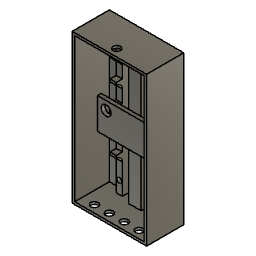
Locker-Button project (Autodesk Fusion 360 design; units mm, degrees)
Autodesk Fusion 360 part; units mm, degrees
note: some values were not read from the file. Chosen so that the rebuilt part matches the saved one: which face or edge a step refers to; where a step ends.
sketch "Schizzo1" plane through (0, 0, 0) normal (0, 1, 0) x (1, 0, 0) in component "Scatola di fissaggio"
  line L0 (-30, -60) -> (30, -60)
  line L1 (30, -60) -> (30, 60)
  line L2 (30, 60) -> (-30, 60)
  line L3 (-30, 60) -> (-30, -60)
  point P0 (0, -60)
  point P1 (-30, 0)
  dimension "d1" = 60
  dimension "d2" = 120
  constraint horizontal L0
  constraint vertical L1
  constraint horizontal L2
  constraint vertical L3
  constraint midpoint L0 P0
  constraint midpoint L3 P1
  constraint vertical origin P0
  constraint horizontal origin P1
  measures "d1" distance of L0.start L0.end
  measures "d2" distance of L0.start L2.end
extrude "Estrusione1" add sketch "Schizzo1" along normal blind 30 makes body 1 in component "Scatola di fissaggio"
shell "Svuotamento1" thickness 2 removed faces 1 at (-10, 0, 20) on bodies 1 in component "Scatola di fissaggio"
ref_plane "Piano di lavoro1" through (0, 14, -58) normal (0, 0, 1) x (1, 0, 0) in component "Guida lineare"
sketch "Schizzo1 (2)" plane through (0, 12.5, -58) normal (0, 0, 1) x (1, 0, 0) in component "Guida lineare"
  line L0 (0, -18.6959) -> (0, 30.9147) construction
  line L1 (0, 8) -> (-5, 8)
  line L2 (-5, 8) -> (-5, 11.5)
  line L3 (-3.5, 13) -> (-2.5, 13)
  line L4 (-2.5, 13) -> (-2.5, 15.5)
  line L5 (28, 15.5) -> (-28, 15.5)
  line L6 (-5, 11.5) -> (-3.5, 13)
  line L7 (0, 8) -> (5, 8)
  line L8 (5, 8) -> (5, 11.5)
  line L9 (5, 11.5) -> (3.5, 13)
  line L10 (3.5, 13) -> (2.5, 13)
  line L11 (2.5, 13) -> (2.5, 15.5)
  point P0 (-5, 13)
  dimension "d7" = 2.5
  dimension "d8" = 5
  dimension "d9" = 5
  dimension "d10" = 2.5
  dimension "d11" = 1.5
  dimension "d12" = 1.5
  constraint vertical L0
  constraint coincident origin L0
  constraint coincident L0 L1.start
  constraint perpendicular L0 L1
  constraint perpendicular L1 L2
  constraint perpendicular L2 L3
  constraint perpendicular L3 L4
  constraint coincident L4.end L5
  constraint coincident P0 L2
  constraint coincident P0 L3
  constraint symmetric L0 L1.start L7.start
  constraint symmetric L0 L1.end L7.end
  constraint symmetric L0 L3.end L10.end
  constraint symmetric L0 L4.end L11.end
  constraint symmetric L0 L2.end L8.end
  constraint symmetric L0 L3.start L9.end
  measures "d7" distance of L3.end L4.end
  measures "d8" distance of L1.end P0
  measures "d9" distance of L1.start L1.end
  measures "d10" distance of L0 L4
  measures "d11" distance of P0 L2.end
  measures "d12" distance of P0 L3.start
extrude "Estrusione1'" add sketch "Schizzo1 (2)" along normal up to near side of body 1 separate body makes body 2 in component "Guida lineare"
sketch "Schizzo5" plane through (0, 0, 0) normal (0, 0, 1) x (1, 0, 0) in component "Base mobile"
  line L0 (5, 24) -> (3.5, 25.5)
  line L1 (5, 20.5) -> (5, 24)
  line L2 (0, 20.5) -> (5, 20.5)
  line L3 (0, 20) -> (5.5, 20)
  line L4 (5.5, 20) -> (5.5, 24.2071)
  line L5 (5.5, 24.2071) -> (3.8536, 25.8536)
  line L6 (3.8536, 25.8536) -> (8.8536, 25.8536)
  line L7 (8.8536, 25.8536) -> (8.8536, 15.8536)
  line L8 (8.8536, 15.8536) -> (0, 15.8536)
  line L9 (0, -6.1959) -> (0, 43.4147)
  line L10 (-8.8536, 15.8536) -> (0, 15.8536)
  line L11 (-8.8536, 25.8536) -> (-8.8536, 15.8536)
  line L12 (0, 20) -> (-5.5, 20)
  line L13 (-5.5, 20) -> (-5.5, 24.2071)
  line L14 (-3.8536, 25.8536) -> (-8.8536, 25.8536)
  line L15 (-5.5, 24.2071) -> (-3.8536, 25.8536)
  dimension "d24" = 0.5
  dimension "d25" = 10
  dimension "d26" = 5
  constraint perpendicular L1 L6
  constraint perpendicular L6 L7
  constraint perpendicular L7 L8
  constraint coincident L8.end L9
  constraint symmetric L3.start L9 L12.start
  constraint symmetric L3.end L9 L12.end
  constraint symmetric L4.end L9 L13.end
  constraint symmetric L5.end L9 L14.start
  constraint symmetric L6.end L9 L11.start
  constraint symmetric L7.end L9 L10.start
  constraint symmetric L8.end L9 L10.end
  measures "d25" distance of L6.end L7.end
  measures "d26" distance of L5.end L6.end
extrude "Estrusione2" add sketch "Schizzo5" along normal blind 5 and the other way blind 5 separate body makes body 3 in component "Base mobile"
sketch "Schizzo6" plane through (0, 15.8536, 0) normal (0, -1, 0) x (1, 0, 0) in component "Base mobile"
  line L0 (8.8536, -5) -> (8.8536, 5)
  line L1 (8.8536, 5) -> (-8.8536, 5)
  line L2 (-8.8536, 5) -> (-8.8536, -5)
  line L3 (-8.8536, -5) -> (8.8536, -5)
  line L4 (22.5, -12.5) -> (-22.5, -12.5)
  line L5 (-22.5, -12.5) -> (-22.5, 12.5)
  line L6 (-22.5, 12.5) -> (22.5, 12.5)
  line L7 (22.5, 12.5) -> (22.5, -12.5)
  point P0 (0, -12.5)
  point P1 (22.5, 0)
  dimension "d31" = 45
  dimension "d32" = 25
  constraint horizontal L4
  constraint vertical L5
  constraint horizontal L6
  constraint vertical L7
  constraint midpoint L4 P0
  constraint midpoint L7 P1
  constraint horizontal origin P1
  constraint vertical origin P0
  measures "d31" distance of L4.start L4.end
  measures "d32" distance of L4.start L6.end
extrude "Estrusione3" add sketch "Schizzo6" along normal blind 3 separate body contours L0 L1 L2 L3 | L4 L5 L6 L7 makes body 4 in component "Base mobile"
sketch "Schizzo1 (3)" plane through (0, 28, 0) normal (0, -1, 0) x (1, 0, 0) in component "cremagliera"
  line L0 (-28, 58) -> (-28, -58)
  line L1 (-28, -58) -> (28, -58)
  line L2 (28, -58) -> (28, 58)
  line L3 (28, 58) -> (-28, 58)
  line L4 (-12.5, -58) -> (-17.5, -58)
  line L5 (-17.5, -58) -> (-17.5, 58)
  line L6 (-17.5, 58) -> (-12.5, 58)
  line L7 (-12.5, 58) -> (-12.5, -58)
  dimension "d35" = 5
  dimension "d36" = 12.5
  constraint horizontal L4
  constraint vertical L5
  constraint horizontal L6
  constraint vertical L7
  constraint collinear L1 L4
  constraint collinear L3 L6
  measures "d35" distance of L4.start L4.end
  measures "d36" distance of origin L7
extrude "Estrusione1''" add sketch "Schizzo1 (3)" along normal blind 10 separate body contours L1 L3 L4 L5 L6 L7 makes body 5 in component "cremagliera"
sketch "Schizzo7" plane through (0, 12.8536, 0) normal (0, -1, 0) x (1, 0, 0) in component "Base mobile"
  line L0 (22.5, 12.5) -> (-22.5, 12.5)
  line L1 (-22.5, 12.5) -> (-22.5, -12.5)
  line L2 (-22.5, -12.5) -> (22.5, -12.5)
  line L3 (22.5, -12.5) -> (22.5, 12.5)
  circle A0 centre (-15.5, 5.5) radius 4
  dimension "d51" = 8
  dimension "d53" = 7
  dimension "d54" = 7
  measures "d51" diameter of A0
  measures "d53" distance of L0 A0.centre
  measures "d54" distance of L1 A0.centre
extrude "Estrusione4" cut sketch "Schizzo7" along normal up to far side of body 4 contours A0 bodies 4 in component "Base mobile"
sketch "Schizzo3" plane through (-17.5, 0, 0) normal (-1, 0, 0) x (0, -1, 0) in component "cremagliera"
  line L0 (-28, 58) -> (-28, -58)
  line L1 (-28, -58) -> (-18, -58)
  line L2 (-18, -58) -> (-18, 58)
  line L3 (-18, 58) -> (-28, 58)
  arc A0 (-18, -29) -> (-23, -34) centre (-18, -34) ccw
  line L4 (-23, -77.8463) -> (-23, -58) construction
  line L5 (-23, -34) -> (-23, 61.2431) construction
  line L6 (-18, -29) -> (-18, -27)
  line L7 (-23, -27) -> (-23, -17)
  line L8 (-18, -27) -> (-23, -27)
  arc A1 (-18, -12) -> (-23, -17) centre (-18, -17) ccw
  line L9 (-18, -12) -> (-18, -10)
  line L10 (-18, -10) -> (-23, -10)
  line L11 (-23, -10) -> (-23, 0)
  arc A2 (-18, 5) -> (-23, 0) centre (-18, 0) ccw
  line L12 (-18, 5) -> (-18, 7)
  line L13 (-23, 7) -> (-18, 7)
  line L14 (-23, 7) -> (-23, 17)
  arc A3 (-18, 22) -> (-23, 17) centre (-18, 17) ccw
  line L15 (-18, 22) -> (-18, 24)
  line L16 (-23, 24) -> (-18, 24)
  line L17 (-23, 24) -> (-23, 34)
  arc A4 (-18, 39) -> (-23, 34) centre (-18, 34) ccw
  line L18 (-18, 39) -> (-18, 41)
  line L19 (-23, 41) -> (-23, 58)
  line L20 (-18, 41) -> (-23, 41)
  line L21 (-23, -34) -> (-23, -58)
  dimension "d57" = 5
  dimension "d58" = 24
  dimension "d59" = 2
  dimension "d60" = 10
  dimension "d61" = 2
  dimension "d62" = 10
  dimension "d63" = 2
  dimension "d64" = 10
  dimension "d65" = 2
  dimension "d66" = 10
  dimension "d67" = 2
  constraint parallel L0 L4
  constraint coincident L2 A0.centre
  constraint tangent A0 L4
  constraint midpoint L1 L4.end
  constraint coincident L2 A0.start
  constraint collinear L4 L5
  constraint coincident L2 L6.end
  constraint parallel L2 L6
  constraint coincident L5 L7.start
  constraint coincident L5 L7.end
  constraint perpendicular L7 L8
  constraint coincident L2 A1.centre
  constraint horizontal L7.end A1.centre
  constraint coincident L2 A1.start
  constraint coincident L2 L9.end
  constraint coincident L5 L10.end
  constraint perpendicular L5 L10
  constraint coincident L5 L11.end
  constraint coincident L2 A2.centre
  constraint horizontal L11.end A2.centre
  constraint coincident L2 A2.start
  constraint coincident L2 L12.end
  constraint parallel L2 L12
  constraint coincident L5 L13.start
  constraint perpendicular L2 L13
  constraint coincident L5 L14.end
  constraint coincident L2 A3.centre
  constraint coincident L14.end A3
  constraint horizontal L14.end A3.centre
  constraint coincident L2 A3.start
  constraint coincident L2 L15.end
  constraint coincident L5 L16.start
  constraint coincident L5 L17.end
  constraint horizontal L16
  constraint coincident L2 A4.centre
  constraint tangent L17 A4
  constraint coincident L2 A4.start
  constraint coincident L2 L18.end
  constraint parallel L2 L18
  constraint coincident L5 L19.start
  constraint midpoint L3 L19.end
  constraint perpendicular L3 L19
  constraint perpendicular L19 L20
  measures "d57" distance of L0 L4
  measures "d58" distance of L1.end A0.centre
  measures "d59" distance of A0.start L6.end
  measures "d60" distance of L7.start L7.end
  measures "d61" distance of A1.start L9.end
  measures "d62" distance of L10.end L11.end
  measures "d63" distance of A2.start L12.end
  measures "d64" distance of L13.start L14.end
  measures "d65" distance of A3.start L15.end
  measures "d66" distance of L16.start L17.end
  measures "d67" distance of A4.start L18.end
extrude "Estrusione3'" cut sketch "Schizzo3" against normal up to surface (5 mm away) contours L2 L3 L19 L20 | L1 L2 A0 L21 | L2 L16 L17 A4 | L2 L7 L8 A1 | L2 L13 L14 A3 | L2 L10 L11 A2 bodies 5 in component "cremagliera"
sketch "Schizzo4" plane through (0, 23, 0) normal (0, -1, 0) x (1, 0, 0) in component "cremagliera"
  line L0 (-12.5, -58) -> (-12.5, -34)
  line L1 (-12.5, -34) -> (-17.5, -34)
  line L2 (-17.5, -34) -> (-17.5, -58)
  line L3 (-17.5, -58) -> (-12.5, -58)
  circle A0 centre (-15, -48) radius 2
  circle A1 centre (-15, 53) radius 2
  line L4 (-17.5, 41) -> (-17.5, 58)
  line L5 (-28, 58) -> (28, 58)
  dimension "d70" = 4
  dimension "d71" = 2.5
  dimension "d72" = 10
  dimension "d73" = 4
  dimension "d74" = 2.5
  dimension "d75" = 5
  measures "d70" diameter of A0
  measures "d71" distance of L2 A0.centre
  measures "d72" distance of L3 A0.centre
  measures "d73" diameter of A1
  measures "d74" distance of A1.centre L4
  measures "d75" distance of A1.centre L5
extrude "Estrusione4'" cut sketch "Schizzo4" against normal up to surface (5 mm away) contours A0 | A1 bodies 5 in component "cremagliera"
sketch "Schizzo2" plane through (0, 0, 0) normal (0, 1, 0) x (1, 0, 0) in component "Scatola di fissaggio"
  circle A0 centre (-15, 48) radius 2
  circle A1 centre (-15, -53) radius 2
extrude "Estrusione2'" cut sketch "Schizzo2" along normal up to surface (30 mm away) bodies 1 in component "Scatola di fissaggio"
sketch "Schizzo3 (2)" plane through (0, 0, 60) normal (0, 0, 1) x (-1, 0, 0) in component "Scatola di fissaggio"
  line L0 (30, 0) -> (-30, 0)
  line L1 (-30, 0) -> (-30, -30)
  line L2 (-30, -30) -> (30, -30)
  line L3 (30, -30) -> (30, 0)
  circle A0 centre (0, -6) radius 3
  dimension "d82" = 6
  dimension "d83" = 6
  constraint vertical origin A0.centre
  measures "d82" diameter of A0
  measures "d83" distance of L0 A0.centre
extrude "Estrusione3''" cut sketch "Schizzo3 (2)" against normal up to surface (2 mm away) contours A0 bodies 1 in component "Scatola di fissaggio"
sketch "Schizzo4 (2)" plane through (0, 0, -60) normal (0, 0, -1) x (1, 0, 0) in component "Scatola di fissaggio"
  line L0 (30, 0) -> (-30, 0)
  line L1 (-30, 0) -> (-30, -30)
  line L2 (-30, -30) -> (30, -30)
  line L3 (30, -30) -> (30, 0)
  circle A0 centre (-18, -6) radius 3
  line L4 (-68.094, -6) -> (66.0156, -6) construction
  line L5 (0, 54.335) -> (0, -66.5386) construction
  circle A1 centre (-6, -6) radius 3
  circle A2 centre (18, -6) radius 3
  circle A3 centre (6, -6) radius 3
  dimension "d86" = 6
  dimension "d91" = 12
  dimension "d92" = 6
  dimension "d93" = 6
  dimension "d94" = 12
  dimension "d97" = 12
  constraint perpendicular L3 L4
  constraint perpendicular L0 L5
  constraint coincident A0.centre L4
  constraint coincident L4 A1.centre
  constraint symmetric A0 L5 A2
  constraint symmetric L5 A1 A3
  measures "d86" diameter of A0
  measures "d91" distance of L1 A0.centre
  measures "d92" distance of L0 L4
  measures "d93" diameter of A1
  measures "d94" distance of A0.centre A1.centre
  measures "d97" distance of L3 A2.centre
extrude "Estrusione4''" cut sketch "Schizzo4 (2)" against normal up to surface (2 mm away) contours A0 | A1 | A2 | A3 bodies 1 in component "Scatola di fissaggio"
component "Scatola di fissaggio" placed x (1, 0, 0) y (0, 1, 0) z (0, 0, 1) at (0, 0, 0)
component "Guida lineare" placed x (1, 0, 0) y (0, 1, 0) z (0, 0, 1) at (0, 0, 0)
component "Base mobile" placed x (1, 0, 0) y (0, 1, 0) z (0, 0, 1) at (0, 0, 0)
component "cremagliera" placed x (1, 0, 0) y (0, 1, 0) z (0, 0, 1) at (0, 0, 0)
equation "d12 = d11"
